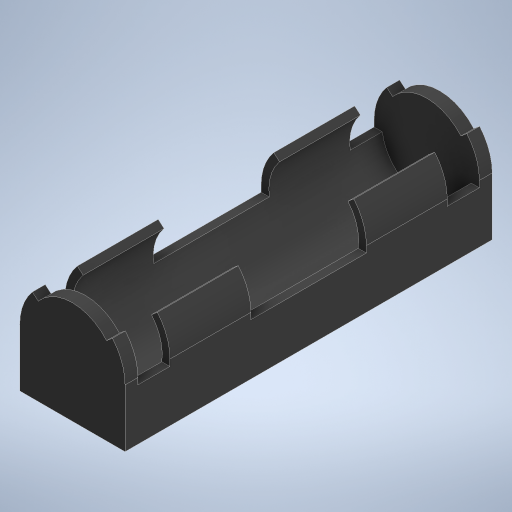
# Autodesk Inventor part: AA_battery_box
Saved by Autodesk Inventor 2024.1 (Build 281209000, 209)
## iProperties
Created: 2025-02-19
Part Number: AA_battery_box
Material: 一般
Document SubType Name: Modeling
Designer: hibik
Density: 1 g/cm^3
Appearance: 既定
Author: hibik
Autodesk Inventor part; units mm, degrees
ref_plane "YZ Plane" through (0, 0, 0) normal (1, 0, 0) x (0, 1, 0)
ref_plane "XZ Plane" through (0, 0, 0) normal (0, 1, 0) x (-1, 0, 0)
ref_plane "XY Plane" through (0, 0, 0) normal (0, 0, 1) x (1, 0, 0)
sketch "スケッチ1" plane through (0, 0, 0) normal (0, 1, 0) x (-1, 0, 0)
  line L0 (8.2, 28.6) -> (-8.2, 28.6)
  line L1 (-8.2, 28.6) -> (-8.2, -28.6)
  line L2 (-8.2, -28.6) -> (8.2, -28.6)
  line L3 (8.2, -28.6) -> (8.2, 28.6)
  line L4 (7, 26.6) -> (-7, 26.6)
  line L5 (-7, 26.6) -> (-7, -26.6)
  line L6 (-7, -26.6) -> (7, -26.6)
  line L7 (7, -26.6) -> (7, 26.6)
  point P0 (0, 0)
  point P1 (8.2, 0)
  point P2 (0, 28.6)
  point P3 (0, 26.6)
  point P4 (7, 0)
  dimension "d0" = 57.2
  dimension "d1" = 16.4
  dimension "d4" = 2
  dimension "d7" = 14
  constraints: 16 end point, 4 midpoint, 4 parallel, 2 horizontal, 2 horizontal alignment, 2 perpendicular, 2 vertical alignment
  measures "d0" distance of L1.end L0.end
  measures "d1" distance of L1.end L2.end
  measures "d4" distance between parallel lines of L0 L4
  measures "d7" distance of L4.start L4.end
extrude "押し出し1" add sketch "スケッチ1" along normal blind 14
sketch "スケッチ2" plane through (-8.2, 0, 28.6) normal (0, 0, 1) x (1, 0, 0)
  circle A0 centre (8.2, 7) radius 7
  line L0 (0, 14) -> (16.4, 14) projected
  line L1 (0, 0) -> (16.4, 0) projected
  circle A1 centre (8.2, 7) radius 8.2
  line L2 (16.4, 0) -> (16.4, 14) projected
  line L3 (8.2, 7) -> (0, 14)
  line L4 (16.4, 14) -> (8.2, 7)
  line L5 (0, 0) -> (0, 14) projected
  point P0 (8.2, 0)
  point P1 (8.2, 0)
  point P2 (2.876, 11.5448)
  point P3 (1.9634, 12.324)
  point P4 (0, 7)
  point P5 (8.2, 0)
  point P6 (14.4366, 12.324)
  point P7 (13.524, 11.5448)
  point P8 (16.4, 7)
  point P9 (8.2, 14)
  dimension "d8" = 14
  constraints: 4 end point, 2 centre point, 2 tangent, 1 coincident, 1 midpoint, 1 vertical alignment
  measures "d8" diameter of A0
extrude "押し出し2" add sketch "スケッチ2" against normal up to surface (57.2 mm away) contours A0 L4 A1 L1 | L1 A1 L3 A0 | L1 L5 A1 | A1 L2 L1
extrude "押し出し3" cut sketch "スケッチ2" against normal through all contours A0 L0 A1 L4 | A0 L3 A1 L0 | L4 L2 A1 | A1 L0 L4 | A1 L3 L0 | A1 L5 L3
sketch "スケッチ3" plane through (0, 0, 0) normal (1, 0, 0) x (0, 1, 0)
  line L0 (0, 26.6) -> (11.5448, 26.6) projected
  line L1 (11.5448, -26.6) -> (11.5448, -26.6) projected
  line L2 (11.5448, -26.6) -> (0, -26.6) projected
  line L3 (0, -26.6) -> (11.5448, -26.6) projected
  line L4 (11.5448, 26.6) -> (11.5448, 26.6) projected
  line L5 (11.5448, 26.6) -> (0, 26.6) projected
  line L6 (0, 26.6) -> (11.5448, 26.6) projected
  line L7 (11.5448, 26.6) -> (14, 26.6) projected
  line L8 (14, -26.6) -> (11.5448, -26.6) projected
  line L9 (-2.8, 0) -> (16.8, 0) projected
  line L10 (14, 9) -> (6, 9)
  line L11 (6, 9) -> (6, -9)
  line L12 (6, -9) -> (14, -9)
  line L13 (14, 26.6) -> (6, 26.6)
  line L14 (6, 26.6) -> (6, 21.6)
  line L15 (6, 21.6) -> (14, 21.6)
  line L16 (14, 21.6) -> (14, 26.6)
  line L17 (14, -26.6) -> (6, -26.6)
  line L18 (6, -26.6) -> (6, -21.6)
  line L19 (6, -21.6) -> (14, -21.6)
  line L20 (14, -21.6) -> (14, -26.6)
  line L21 (14, 9) -> (14, -9)
  line L22 (0, 26.6) -> (0, -26.6) projected
  point P0 (0, 0)
  point P1 (12.7724, -26.6)
  point P2 (14, 0)
  point P3 (0, 0)
  dimension "d13" = 8
  dimension "d14" = 18
  dimension "d15" = 5
  constraints: 24 end point, 5 parallel, 3 equal length, 3 horizontal, 3 midpoint, 3 perpendicular, 1 collinear, 1 horizontal alignment, 1 vertical
  measures "d13" distance of L18.end L19.end
  measures "d14" distance of L10.start L12.end
  measures "d15" distance of L15.end L7.end
extrude "押し出し4" cut sketch "スケッチ3" along normal through all both and the other way through all
sketch "スケッチ4" plane through (0, 0, 0) normal (0, -1, 0) x (1, 0, 0)
  line L0 (-8.2, 28.6) -> (8.2, 28.6) projected
  line L1 (8.2, 28.6) -> (-8.2, 28.6)
  line L2 (-8.2, 28.6) -> (-8.2, -28.6)
  line L3 (-8.2, -28.6) -> (8.2, -28.6)
  line L4 (8.2, -28.6) -> (8.2, 28.6)
  point P0 (0, 0)
  constraints: 8 end point, 2 parallel, 1 coincident, 1 horizontal, 1 perpendicular
extrude "押し出し5" add sketch "スケッチ4" along normal blind 2
